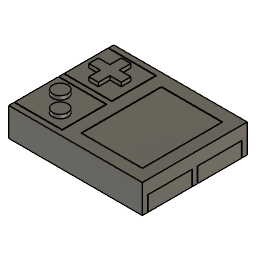
mockup (Autodesk Fusion 360 design; units mm, degrees)
Autodesk Fusion 360 part; units mm, degrees
note: some values were not read from the file. Set by a fixed rule: which face or edge a step refers to.
sketch "Sketch1" plane through (0, 0, 0) normal (0, 0, 1) x (1, 0, 0) in component "Body"
  line L0 (-35, 27.5) -> (35, 27.5)
  line L1 (35, 27.5) -> (35, -27.5)
  line L2 (35, -27.5) -> (-35, -27.5)
  line L3 (-35, -27.5) -> (-35, 27.5)
  point P0 (0, -27.5)
  point P1 (-35, 0)
  dimension "d1" = 55
  dimension "d2" = 70
  constraint horizontal L0
  constraint vertical L1
  constraint horizontal L2
  constraint vertical L3
  constraint midpoint L2 P0
  constraint midpoint L3 P1
  constraint horizontal origin P1
  constraint vertical origin P0
  measures "d1" distance of L0.start L2.end
  measures "d2" distance of L1.end L2.end
extrude "Extrude1" add sketch "Sketch1" along normal blind 15 makes body 1 in component "Body"
sketch "Sketch2" plane through (0, 0, 15) normal (0, 0, 1) x (-1, 0, 0) in component "Body"
  line L0 (-35, -27.5) -> (35, -27.5)
  line L1 (35, -27.5) -> (35, 27.5)
  line L2 (-28.5, 21) -> (3.5, 21)
  line L3 (3.5, 21) -> (3.5, -21)
  line L4 (3.5, -21) -> (-28.5, -21)
  line L5 (-28.5, -21) -> (-28.5, 21)
  line L6 (35, 27.5) -> (-35, 27.5) construction
  line L7 (-35, 27.5) -> (-35, -27.5) construction
  line L8 (-35, -27.5) -> (35, -27.5) construction
  line L9 (-35, 0) -> (0, 0) construction
  line L10 (-28.5, 21) -> (-28.5, 27.5) construction
  line L11 (-28.5, 21) -> (-35, 21) construction
  dimension "d5" = 32
  dimension "d6" = 42
  constraint horizontal L2
  constraint vertical L3
  constraint horizontal L4
  constraint vertical L5
  constraint midpoint L7 L9.start
  constraint coincident L9.end origin
  constraint symmetric L2.start L4.end L9
  constraint coincident L6 L10.end
  constraint perpendicular L6 L10
  constraint coincident L7 L11.end
  constraint perpendicular L7 L11
  constraint equal L10 L11
  measures "d5" distance of L2.start L2.end
  measures "d6" distance of L2.start L4.end
extrude "Extrude2" cut sketch "Sketch2" against normal blind 0.2 bodies 1 in component "Body"
sketch "Sketch3" plane through (0, 0, 15) normal (0, 0, 1) x (-1, 0, 0) in component "Body"
  line L0 (3.5, 21) -> (3.5, -21)
  line L1 (3.5, -21) -> (-28.5, -21)
  line L2 (-28.5, -21) -> (-28.5, 21)
  line L3 (-28.5, 21) -> (3.5, 21)
  line L4 (35, 27.5) -> (-35, 27.5)
  line L5 (-35, 27.5) -> (-35, -27.5)
  line L6 (-35, -27.5) -> (35, -27.5)
  line L7 (35, -27.5) -> (35, 27.5)
  line L8 (35, -24.5) -> (10, -24.5)
  line L9 (10, -24.5) -> (10, -1.5)
  line L10 (10, -1.5) -> (35, -1.5)
  line L11 (35, -1.5) -> (35, -24.5)
  line L12 (35, 0) -> (35, -1.5) construction
  line L13 (35, -24.5) -> (35, -26) construction
  line L14 (35, -26) -> (35, -27.5) construction
  dimension "d9" = 23
  dimension "d10" = 25
  constraint horizontal L8
  constraint vertical L9
  constraint horizontal L10
  constraint vertical L11
  constraint coincident L7 L8.start
  constraint midpoint L7 L12.start
  constraint coincident L7 L13.end
  constraint coincident L6.end L7.start
  constraint equal L13 L14
  constraint equal L12 L13
  measures "d9" distance of L8.start L10.end
  measures "d10" distance of L8.start L8.end
extrude "Extrude3" cut sketch "Sketch3" against normal blind 8 contours L7 L8 L9 L10 L11 bodies 1 in component "Body"
mirror "Mirror1" about plane through (0, 0, 0) normal (0, 1, 0) of "Extrude3" in component "Body"
sketch "Sketch4" plane through (0, 0, 0) normal (0, 0, -1) x (1, 0, 0) in component "Body"
  line L0 (35, 27.5) -> (-35, 27.5)
  line L1 (-35, 27.5) -> (-35, -27.5)
  line L2 (-35, -27.5) -> (35, -27.5)
  line L3 (35, -27.5) -> (35, 27.5)
  line L4 (-10, 1.5) -> (-35, 1.5) construction
  line L5 (-35, 1.5) -> (-35, 24.5) construction
  line L6 (-35, 24.5) -> (-10, 24.5) construction
  line L7 (-10, 24.5) -> (-10, 1.5) construction
  line L8 (35, 1.5) -> (10, 1.5)
  line L9 (10, 1.5) -> (10, 24.5)
  line L10 (10, 24.5) -> (35, 24.5)
  line L11 (35, 24.5) -> (35, 1.5)
  constraint horizontal L8
  constraint vertical L9
  constraint horizontal L10
  constraint vertical L11
  constraint coincident L3 L8.start
  constraint equal L7 L9
  constraint equal L6 L10
  constraint horizontal L6.end L9.end
extrude "Extrude4" cut sketch "Sketch4" against normal blind 8 contours L3 L8 L9 L10 L11 bodies 1 in component "Body"
mirror "Mirror2" about plane through (0, 0, 0) normal (0, 1, 0) of "Extrude4" in component "Body"
sketch "Sketch1 (2)" plane through (0, 0, 7) normal (0, 0, 1) x (-1, 0, 0) in component "DPad"
  line L0 (35, -1.5) -> (10, -1.5)
  line L1 (10, -1.5) -> (10, -24.5)
  line L2 (10, -24.5) -> (35, -24.5)
  line L3 (35, -24.5) -> (35, -1.5)
extrude "Extrude1'" add sketch "Sketch1 (2)" along normal blind 8 separate body makes body 2 in component "DPad"
sketch "Sketch2 (2)" plane through (0, 0, 15) normal (0, 0, 1) x (-1, 0, 0) in component "DPad"
  line L0 (35, -24.5) -> (35, -1.5)
  line L1 (35, -1.5) -> (10, -1.5)
  line L2 (10, -1.5) -> (10, -24.5)
  line L3 (10, -24.5) -> (35, -24.5)
  line L4 (25, -15.5) -> (25, -21.5)
  line L5 (25, -21.5) -> (20, -21.5)
  line L6 (20, -21.5) -> (20, -15.5)
  line L7 (20, -15.5) -> (14, -15.5)
  line L8 (14, -15.5) -> (14, -10.5)
  line L9 (14, -10.5) -> (20, -10.5)
  line L10 (20, -10.5) -> (20, -4.5)
  line L11 (20, -4.5) -> (25, -4.5)
  line L12 (25, -4.5) -> (25, -10.5)
  line L13 (25, -10.5) -> (31, -10.5)
  line L14 (31, -10.5) -> (31, -15.5)
  line L15 (31, -15.5) -> (25, -15.5)
  line L16 (25, -15.5) -> (20, -15.5) construction
  line L17 (20, -15.5) -> (20, -10.5) construction
  line L18 (22.5, -13) -> (22.5, -15.5) construction
  line L19 (22.5, -13) -> (20, -13) construction
  line L20 (10, -24.5) -> (35, -1.5) construction
  line L21 (35, -24.5) -> (10, -1.5) construction
  point P0 (22.5, -15.5)
  point P1 (20, -13)
  point P2 (22.5, -13)
  point P3 (22.5, -13)
  dimension "d22" = 5
  dimension "d23" = 6
  constraint perpendicular L3 L4
  constraint perpendicular L4 L5
  constraint perpendicular L5 L6
  constraint perpendicular L6 L7
  constraint perpendicular L7 L8
  constraint perpendicular L8 L9
  constraint perpendicular L9 L10
  constraint perpendicular L10 L11
  constraint perpendicular L11 L12
  constraint perpendicular L12 L13
  constraint perpendicular L13 L14
  constraint horizontal L15
  constraint equal L5 L8
  constraint equal L8 L11
  constraint equal L11 L14
  constraint equal L6 L9
  constraint equal L9 L12
  constraint equal L12 L15
  constraint horizontal L16
  constraint vertical L17
  constraint midpoint L16 P0
  constraint midpoint L17 P1
  constraint coincident P3 P2
  constraint coincident P0 L18.end
  constraint coincident L17 P1
  constraint perpendicular L17 L19
  constraint vertical L18
  constraint coincident P1 L19.end
  constraint coincident L2.end L3.start
  constraint coincident L0.end L1.start
  constraint coincident L0.start L3.end
  constraint coincident L1.end L2.start
  constraint coincident L20 P3
  constraint coincident L21 P3
  measures "d22" distance of L4.end L5.end
  measures "d23" distance of L5.end L6.end
extrude "Extrude2'" add sketch "Sketch2 (2)" along normal blind 2 contours L4 L5 L6 L7 L8 L9 L10 L11 L12 L13 L14 L15 bodies 2 in component "DPad"
sketch "Sketch1 (3)" plane through (0, 0, 7) normal (0, 0, 1) x (-1, 0, 0) in component "AB"
  line L0 (10, 1.5) -> (35, 1.5)
  line L1 (35, 1.5) -> (35, 24.5)
  line L2 (35, 24.5) -> (10, 24.5)
  line L3 (10, 24.5) -> (10, 1.5)
extrude "Extrude1''" add sketch "Sketch1 (3)" along normal blind 8 separate body makes body 3 in component "AB"
sketch "Sketch2 (3)" plane through (0, 0, 15) normal (0, 0, 1) x (-1, 0, 0) in component "AB"
  line L0 (10, 24.5) -> (10, 1.5)
  line L1 (10, 1.5) -> (35, 1.5)
  line L2 (35, 1.5) -> (35, 24.5)
  line L3 (35, 24.5) -> (10, 24.5)
  circle A0 centre (18.2574, 17.2426) radius 4
  circle A1 centre (26.7426, 8.7574) radius 4
  line L4 (18.2574, 17.2426) -> (26.7426, 8.7574) construction
  line L5 (35, 24.5) -> (10, 1.5) construction
  line L6 (10, 24.5) -> (35, 1.5) construction
  point P0 (22.5, 13)
  dimension "d29" = 45
  dimension "d31" = 8
  dimension "d32" = 12
  constraint equal A0 A1
  constraint coincident A0.centre L4.start
  constraint coincident A1.centre L4.end
  constraint midpoint L4 P0
  constraint coincident L2.end L3.start
  constraint coincident L0.end L1.start
  constraint coincident L0.start L3.end
  constraint coincident L1.end L2.start
  constraint coincident P0 L5
  constraint coincident P0 L6
  measures "d29" angle of L1 L4
  measures "d31" diameter of A0
  measures "d32" distance of A0.centre A1.centre
extrude "Extrude2''" add sketch "Sketch2 (3)" along normal blind 2 contours A0 | A1 bodies 3 in component "AB"
extrude "Extrude1'''" add 1 faces at (18.3333, -16.8333, 8) along direction (0, 0, -1) blind 8 separate body on bodies 1 makes body 4 in component "BackA"
extrude "Extrude1''''" add 1 faces at (18.3333, 16.8333, 8) along direction (0, 0, -1) blind 8 separate body on bodies 1 makes body 5 in component "BackB"
move_face "OffsetFaces1" offset -0.2 12 faces at (-26.6667, 24.5, 12.3333) (-10, 16.8333, 12.3333) (-18.3333, 1.5, 12.3333) (-18.3333, -1.5, 12.3333) (-10, -16.8333, 12.3333) (-26.6667, -24.5, 12.3333) (10, 9.1667, 2.6667) (18.3333, 24.5, 2.6667) (26.6667, 1.5, 2.6667) (26.6667, -1.5, 2.6667) (10, -9.1667, 2.6667) (18.3333, -24.5, 2.6667) on bodies 1 in component "Body"
component "Body" placed x (1, 0, 0) y (0, 1, 0) z (0, 0, 1) at (0, 0, 0)
component "DPad" placed x (1, 0, 0) y (0, 1, 0) z (0, 0, 1) at (0, 0, 0)
component "AB" placed x (1, 0, 0) y (0, 1, 0) z (0, 0, 1) at (0, 0, 0)
component "BackA" placed x (1, 0, 0) y (0, 1, 0) z (0, 0, 1) at (0, 0, 0)
component "BackB" placed x (1, 0, 0) y (0, 1, 0) z (0, 0, 1) at (0, 0, 0)
